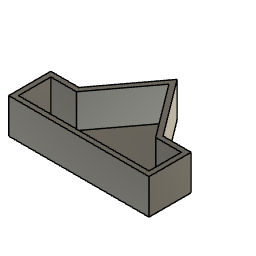
base v1 (Autodesk Fusion 360 design; units mm, degrees)
Autodesk Fusion 360 part; units mm, degrees
sketch "Boceto1" plane through (0, 0, 0) normal (0, 1, 0) x (1, 0, 0)
  line L0 (-50, -40) -> (-50, 0)
  line L1 (-50, 0) -> (80, 0)
  line L2 (80, 0) -> (80, -40)
  line L3 (80, -40) -> (10, -100)
  line L4 (10, -100) -> (-50, -40)
  constraint vertical L0
  constraint perpendicular L0 L1
  constraint perpendicular L1 L2
sketch "Boceto2" plane through (0, 0, 0) normal (0, 0, 1) x (1, 0, 0)
  line L0 (-50.5346, -0.7995) -> (-50.5346, -60.7995)
  line L1 (-50.5346, -60.7995) -> (149.4654, -60.7995)
  line L2 (149.4654, -60.7995) -> (149.4654, -0.7995)
  line L3 (149.4654, -0.7995) -> (109.4654, -0.7995)
  line L4 (109.4654, -0.7995) -> (49.4654, 79.2005)
  line L5 (49.4654, 79.2005) -> (-10.5346, -0.7995)
  line L6 (-10.5346, -0.7995) -> (-50.5346, -0.7995)
  dimension "d4" = 200
  dimension "d5" = 60
  dimension "d6" = 40
  dimension "d7" = 40
  dimension "d8" = 100
  dimension "d9" = 100
  dimension "d10" = 60
  constraint vertical L0
  constraint perpendicular L0 L1
  constraint perpendicular L1 L2
  constraint perpendicular L0 L3
  constraint perpendicular L0 L6
  measures "d4" distance of L0.end L1.end
  measures "d5" distance of L0.start L0.end
  measures "d6" distance of L0.start L5.end
  measures "d7" distance of L2.end L3.end
  measures "d8" distance of L3.end L4.end
  measures "d9" distance of L4.end L5.end
  measures "d10" distance of L1.end L2.end
extrude "Extruir2" add sketch "Boceto2" along normal blind 50
shell "Vaciado2" thickness 7 removed faces 1 at (49.4654, 25.8671, 50)
sketch "Boceto3" plane through (0, 0, 7) normal (0, 0, 1) x (-1, 0, 0)
  line L0 (7.0346, 7.7995) -> (43.5346, 7.7995)
  line L1 (43.5346, 7.7995) -> (43.5346, 53.7995)
  line L2 (43.5346, 53.7995) -> (-142.4654, 53.7995)
  line L3 (-142.4654, 53.7995) -> (-142.4654, 7.7995)
  line L4 (-142.4654, 7.7995) -> (-105.9654, 7.7995)
  line L5 (-105.9654, 7.7995) -> (-49.4654, -67.5338)
  line L6 (-49.4654, -67.5338) -> (7.0346, 7.7995)
sketch "Boceto4" plane through (0, 0, 7) normal (0, 0, 1) x (-1, 0, 0)
  line L0 (45, 50) -> (35, 50)
  line L1 (35, 50) -> (35, 10)
  line L2 (35, 10) -> (45, 10)
  line L3 (45, 10) -> (45, 50)
  constraint horizontal L0
  constraint vertical L1
  constraint horizontal L2
  constraint vertical L3
extrude "Extruir3" cut sketch "Boceto4" sketch "Boceto3" against normal blind 5 of sketch 2
